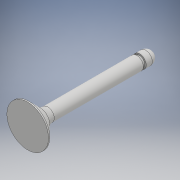
# Autodesk Inventor part: Component 24 (Valve)
Saved by Autodesk Inventor 2018 (Build 220112000, 112)
## iProperties
Created: 2023-03-25
Part Number: Component 24 (Valve)
Material: Generic
Document SubType Name: Modeling
Designer: Habib Mohamed
Density: 1 g/cm^3
Appearance: Default
Author: Habib Mohamed
Autodesk Inventor part; units mm, degrees
ref_plane "YZ Plane" through (0, 0, 0) normal (1, 0, 0) x (0, 1, 0)
ref_plane "XZ Plane" through (0, 0, 0) normal (0, 1, 0) x (-1, 0, 0)
ref_plane "XY Plane" through (0, 0, 0) normal (0, 0, 1) x (1, 0, 0)
sketch "Sketch1" plane through (0, 0, 0) normal (1, 0, 0) x (0, 1, 0)
  line L0 (0, 0) -> (28.5, 0)
  line L1 (24.95, 1.5) -> (4.5855, 1.5)
  line L2 (2.8178, 2.2322) -> (0.3, 4.75)
  line L3 (0.3, 4.75) -> (0, 4.75)
  line L4 (0, 4.75) -> (0, 0)
  arc A0 (28.5, 0) -> (27, 1.5) centre (27, 0) ccw
  line L5 (24.95, 1.5) -> (24.95, 1.15)
  line L6 (24.95, 1.15) -> (25.6, 1.15)
  line L7 (25.6, 1.15) -> (25.6, 1.5)
  line L8 (25.6, 1.5) -> (27, 1.5)
  arc A1 (2.8178, 2.2322) -> (4.5855, 1.5) centre (4.5855, 4) ccw
  dimension "d1" = 4.75
  dimension "d2" = 1.5
  dimension "d3" = 0.3
  dimension "d4" = 45
  dimension "d5" = 1.5
  dimension "d6" = 1.15
  dimension "d8" = 0.65
  dimension "d9" = 1.4
  dimension "d10" = 27
  dimension "d11" = 2.5
  constraints: 18 end point, 4 perpendicular, 4 point on circle, 2 centre point, 2 tangent, 1 collinear, 1 horizontal, 1 parallel, 1 point on line, 1 vertical
  measures "d1" distance of L3.end L0.start
  measures "d2" radius of A0
  measures "d3" distance of L3.end L2.end
  measures "d4" angle of L4 L2
  measures "d5" distance between parallel lines of L0 L1
  measures "d6" distance between parallel lines of L6 L0
  measures "d8" distance of L5.end L6.end
  measures "d9" distance of L7.end L8.end
  measures "d10" distance from line of L4 L8.end
  measures "d11" radius of A1
revolve "Revolution1" add sketch "Sketch1" angle 360 about axis through (0, 0, 0) along (0, 1, 0)
body "Solid1"
